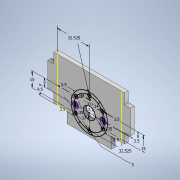
# Autodesk Inventor part: pump part
Saved by Autodesk Inventor 2022 (Build 260153000, 153)
## iProperties
Created: 2022-04-11
Part Number: pump part
Material: Generic
Document SubType Name: Modeling
Designer: j.trilleras
Density: 1 g/cm^3
Appearance: Default
Author: j.trilleras
Autodesk Inventor part; units mm, degrees
ref_plane "YZ Plane" through (0, 0, 0) normal (1, 0, 0) x (0, 1, 0)
ref_plane "XZ Plane" through (0, 0, 0) normal (0, 1, 0) x (-1, 0, 0)
ref_plane "XY Plane" through (0, 0, 0) normal (0, 0, 1) x (1, 0, 0)
sketch "Sketch1" plane through (0, 0, 0) normal (0, 0, 1) x (1, 0, 0)
  line L0 (-22.1985, -10.6442) -> (22.8515, -10.6442)
  line L1 (22.8515, -10.6442) -> (22.8515, 0.6058)
  line L2 (22.8515, 0.6058) -> (32.8515, 0.6058)
  line L3 (32.8515, 0.6058) -> (32.8515, 45.6058)
  line L4 (32.8515, 45.6058) -> (-32.1985, 45.6058)
  line L5 (-32.1985, 45.6058) -> (-32.1985, 0.6058)
  line L6 (-32.1985, 0.6058) -> (-22.1985, 0.6058)
  line L7 (-22.1985, 0.6058) -> (-22.1985, -10.6442)
  point P0 (0, 0)
  dimension "d0" = 45.05
  dimension "d1" = 11.25
  dimension "d2" = 10
  dimension "d3" = 45
  dimension "d4" = 45
  dimension "d5" = 10
  dimension "d6" = 65.05
  constraints: 16 end point, 5 perpendicular, 1 horizontal, 1 parallel
  measures "d0" distance of L0.start L0.end
  measures "d1" distance of L0.end L1.end
  measures "d2" distance of L1.end L2.end
  measures "d3" distance of L2.end L3.end
  measures "d4" distance of L4.end L5.end
  measures "d5" distance of L5.end L6.end
  measures "d6" distance of L3.end L4.end
extrude "Extrusion1" add sketch "Sketch1" against normal blind 3.7
sketch "Sketch2" plane through (0, 0, 0) normal (0, 0, 1) x (1, 0, 0)
  point P0 (0, 0)
sketch "Sketch3" plane through (0, 0, 0) normal (0, 0, 1) x (1, 0, 0)
  circle A0 centre (0.3265, 10.1058) radius 6.05
  line L0 (-32.1985, 45.6058) -> (-32.1985, 0.6058) projected
  line L1 (-32.1985, 0.6058) -> (-22.1985, 0.6058) projected
  circle A1 centre (14.3265, 10.1058) radius 3.175
  circle A2 centre (-13.6735, 10.1058) radius 3.175
  circle A3 centre (0.3265, 10.1058) radius 15.5
  circle A4 centre (0.3265, 25.6058) radius 1.75
  circle A5 centre (0.3265, -5.3942) radius 1.5
  line L2 (32.8515, 0.6058) -> (32.8515, 45.6058) projected
  circle A6 centre (-12.9494, 18.1058) radius 1.75
  circle A7 centre (-13.5028, 3.1058) radius 1.75
  circle A8 centre (14.1558, 3.1058) radius 1.75
  circle A9 centre (13.6024, 18.1058) radius 1.75
  circle A10 centre (0.3265, 10.1058) radius 18.5
  point P0 (0, 0)
  dimension "d9" = 12.1
  dimension "d10" = 32.525
  dimension "d11" = 9.5
  dimension "d12" = 6.35
  dimension "d13" = 14
  dimension "d14" = 6.35
  dimension "d15" = 14
  dimension "d20" = 31
  dimension "d21" = 3.5
  dimension "d22" = 32.525
  dimension "d23" = 3
  dimension "d24" = 32.525
  dimension "d25" = 3.5
  dimension "d26" = 8
  dimension "d27" = 3.5
  dimension "d28" = 3.5
  dimension "d29" = 3.5
  dimension "d30" = 8
  dimension "d31" = 15
  dimension "d36" = 37
  dimension "d54" = 15
  constraints: 11 centre point, 6 point on circle, 2 coincident
  measures "d9" diameter of A0
  measures "d10" distance from line of L0 A0.centre
  measures "d11" distance from line of A0.centre L1
  measures "d12" diameter of A1
  measures "d13" distance of A0.centre A1.centre
  measures "d14" diameter of A2
  measures "d15" distance of A0.centre A2.centre
  measures "d20" diameter of A3
  measures "d21" diameter of A4
  measures "d22" distance from line of L0 A4.centre
  measures "d23" diameter of A5
  measures "d24" distance from line of L2 A5.centre
  measures "d25" diameter of A6
  measures "d26" vertical distance of A0.centre A6.centre
  measures "d27" diameter of A7
  measures "d28" diameter of A8
  measures "d29" diameter of A9
  measures "d30" vertical distance of A3.centre A9.centre
  measures "d31" vertical distance of A8.centre A9.centre
  measures "d36" diameter of A10
  measures "d54" vertical distance of A7.centre A6.centre
extrude "Extrusion2" cut sketch "Sketch3" against normal blind 5 contours A0
sketch "Sketch4" plane through (0, 0, 0) normal (0, 0, 1) x (1, 0, 0)
  point P0 (0, 0)
extrude "Extrusion4" cut sketch "Sketch3" against normal blind 3.5 contours A1 A3 | A3 A1 | A3 A2 | A2 A3
extrude "Extrusion5" cut sketch "Sketch3" against normal blind 5 contours A9 A3 | A3 A9 | A8 A3 | A3 A8 | A4 A3 | A3 A4 | A5 A3 | A3 A5 | A6 A3 | A3 A6 | A7 A3 | A3 A7
sketch "Sketch5" plane through (0, 0, 0) normal (0, 0, 1) x (1, 0, 0)
  point P0 (0, 0)
sketch "Sketch6" plane through (0, 0, 0) normal (0, 0, 1) x (1, 0, 0)
  line L0 (-35.5885, 45.6058) -> (-32.1985, 45.6058)
  line L1 (-32.1985, 45.6058) -> (-32.1985, 0.6058)
  line L2 (-32.1985, 0.6058) -> (-35.5885, 0.6058)
  line L3 (-35.5885, 0.6058) -> (-35.5885, 45.6058)
  line L4 (-32.1985, 45.6058) -> (-32.1985, 0.6058) projected
  line L5 (32.8515, 45.6058) -> (-32.1985, 45.6058) projected
  line L6 (-32.1985, 0.6058) -> (-22.1985, 0.6058) projected
  line L7 (32.8515, 45.6058) -> (32.8515, 0.6058)
  line L8 (32.8515, 0.6058) -> (32.8515, 45.6058) projected
  line L9 (32.8515, 0.6058) -> (36.2415, 0.6058)
  line L10 (36.2415, 0.6058) -> (36.2415, 45.6058)
  line L11 (36.2415, 45.6058) -> (32.8515, 45.6058)
  line L12 (22.8515, 0.6058) -> (32.8515, 0.6058) projected
  point P0 (0, 0)
  dimension "d37" = 0
  dimension "d38" = 0
  dimension "d39" = 0
  dimension "d40" = 3.39
  dimension "d41" = 3.39
  dimension "d42" = 0
  dimension "d43" = 0
  dimension "d44" = 0
  constraints: 16 end point, 6 perpendicular, 1 collinear, 1 horizontal
  measures "d37" distance between parallel lines of L4 L1
  measures "d38" distance between parallel lines of L5 L0
  measures "d39" distance between parallel lines of L6 L2
  measures "d40" distance between parallel lines of L3 L1
  measures "d41" distance between parallel lines of L10 L7
  measures "d42" distance between parallel lines of L8 L7
  measures "d43" distance between parallel lines of L5 L11
  measures "d44" distance between parallel lines of L12 L9
extrude "Extrusion6" add sketch "Sketch6" against normal blind 3.7
sketch "Sketch7" plane through (0, 0, 0) normal (0, 0, 1) x (1, 0, 0)
  line L0 (30.309, 35.2858) -> (30.309, 10.9258)
  line L1 (30.309, 10.9258) -> (42.3265, 10.9258)
  line L2 (42.3265, 10.9258) -> (42.3265, 35.2858)
  line L3 (42.3265, 35.2858) -> (30.309, 35.2858)
  line L4 (36.2415, 45.6058) -> (-35.5885, 45.6058) projected
  line L5 (22.8515, 0.6058) -> (36.2415, 0.6058) projected
  line L6 (36.2415, 0.6058) -> (36.2415, 45.6058) projected
  line L7 (-41.6735, 35.2858) -> (-29.8249, 35.2858)
  line L8 (-29.8249, 35.2858) -> (-29.8249, 10.9258)
  line L9 (-29.8249, 10.9258) -> (-41.6735, 10.9258)
  line L10 (-41.6735, 10.9258) -> (-41.6735, 35.2858)
  line L11 (-35.5885, 0.6058) -> (-22.1985, 0.6058) projected
  line L12 (-35.5885, 45.6058) -> (-35.5885, 0.6058) projected
  point P0 (0, 0)
  point P1 (36.2415, 35.2858)
  point P2 (36.2415, 10.9258)
  point P3 (-35.5885, 10.9258)
  point P4 (-35.5885, 35.2858)
  dimension "d47" = 10.32
  dimension "d48" = 10.32
  dimension "d49" = 6.085
  dimension "d50" = 10.32
  dimension "d51" = 6.085
  constraints: 16 end point, 6 perpendicular, 1 horizontal, 1 vertical
  measures "d47" distance between parallel lines of L4 L3
  measures "d48" distance between parallel lines of L5 L1
  measures "d49" distance between parallel lines of L6 L2
  measures "d50" distance between parallel lines of L9 L11
  measures "d51" distance between parallel lines of L12 L10
extrude "Extrusion7" add sketch "Sketch7" against normal blind 3.7 contours L12 L9 L10 L7 | L3 L2 L1 L6
body "Solid1"
